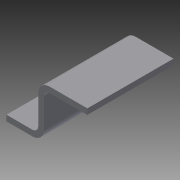
# Autodesk Inventor part: Part6
Saved by Autodesk Inventor 2015 SP1 (Build 190203100, 203)
## iProperties
Created: 2015-04-04
Part Number: Part6
Material: Generic
Document SubType Name: Modeling
Designer: Cyril
Density: 1 g/cm^3
Appearance: Default
Author: Cyril
Autodesk Inventor part; units mm, degrees
ref_plane "YZ Plane" through (0, 0, 0) normal (1, 0, 0) x (0, 1, 0)
ref_plane "XZ Plane" through (0, 0, 0) normal (0, 1, 0) x (-1, 0, 0)
ref_plane "XY Plane" through (0, 0, 0) normal (0, 0, 1) x (1, 0, 0)
sketch "Sketch1" plane through (0, 0, 0) normal (0, 0, 1) x (1, 0, 0)
  line L0 (-0.0319, -2) -> (0.0319, 0)
  line L1 (0.0319, 0) -> (-13.0931, 0)
  line L2 (-33.7741, 0) -> (5.6662, 0) projected
  line L3 (0, -22.7598) -> (0, 4.7598) projected
  line L4 (-0.0319, -2) -> (-13.0931, -2)
  arc A0 (-13.0931, -2) -> (-15.0931, -4) centre (-13.0931, -4) ccw
  line L5 (-15.0931, -4) -> (-15.0931, -14)
  arc A1 (-19.0931, -18) -> (-15.0931, -14) centre (-19.0931, -14) ccw
  line L6 (-19.0931, -18) -> (-28.1398, -18)
  line L7 (-28.1398, -18) -> (-28.1398, -16)
  line L8 (-28.1398, -16) -> (-19.0931, -16)
  arc A2 (-19.0931, -16) -> (-17.0931, -14) centre (-19.0931, -14) ccw
  arc A3 (-13.0931, 0) -> (-17.0931, -4) centre (-13.0931, -4) ccw
  line L9 (-17.0931, -14) -> (-17.0931, -4)
  point P0 (-4.1204, -1.7073)
  point P1 (-27.9684, 0)
  point P2 (0, -1)
  dimension "d4" = 2
  dimension "d5" = 4
  dimension "d6" = 16
  dimension "d7" = 2
  dimension "d9" = 2
  dimension "d10" = 2
  dimension "d11" = 2
  dimension "d12" = 4
  constraints: 16 end point, 8 point on circle, 8 tangent, 4 centre point, 3 perpendicular, 3 point on line, 2 horizontal, 2 vertical, 1 midpoint
  measures "d4" distance of L6.end L7.end
  measures "d5" radius of A3
  measures "d6" distance between parallel lines of L6 L4
  measures "d7" vertical distance of L0.start L0.end
  measures "d9" distance between parallel lines of L9 L5
  measures "d10" radius of A2
  measures "d11" radius of A0
  measures "d12" radius of A1
extrude "Extrusion1" add sketch "Sketch1" along normal blind 30
body "Solid1"
